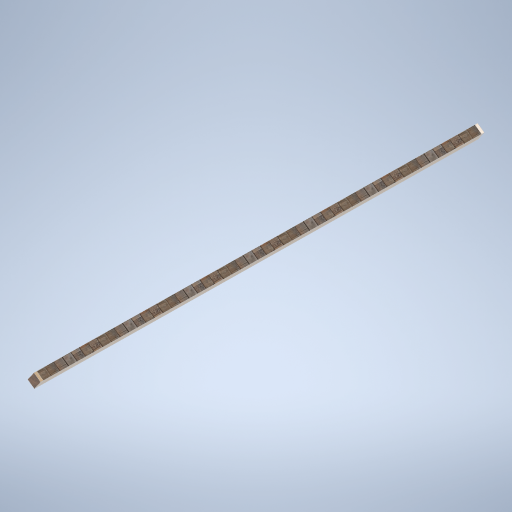
# Autodesk Inventor part: support_beam_segment_0106
Saved by Autodesk Inventor 2024.2 (Build 282272000, 272)
## iProperties
Created: 2024-05-20
Part Number: support_beam_segment_0106
Material: Wood (Maple)
Document SubType Name: Modeling
Designer: LOSTER_1
Density: 0.67 g/cm^3
Appearance: Natural Maple - Glossy Dark Tint
Author: LOSTER_1
Autodesk Inventor part; units mm, degrees
ref_plane "YZ Plane" through (0, 0, 0) normal (1, 0, 0) x (0, 1, 0)
ref_plane "XZ Plane" through (0, 0, 0) normal (0, 1, 0) x (-1, 0, 0)
sketch "Sketch1" plane through (0, 0, 0) normal (0, 0, 1) x (1, 0, 0)
  line L0 (-26.862, 36.8638) -> (-141.5773, -126.9666)
  line L1 (96.5672, -49.5284) -> (-26.3079, 36.5048)
  line L2 (-141.5773, -126.9666) -> (-18.7045, -213.0031) construction
  line L3 (-18.1437, -213.3618) -> (96.5672, -49.5284)
  line L4 (96.0404, -49.1304) -> (-18.7045, -213.0031)
  line L5 (-18.7045, -213.0031) -> (-141.5773, -126.9666)
  line L6 (-141.5773, -126.9666) -> (-26.8324, 36.9061)
  line L7 (-26.8324, 36.9061) -> (96.0404, -49.1304)
  line L8 (96.0404, -49.1304) -> (-141.5773, -126.9666) construction
  line L9 (-18.7045, -213.0031) -> (-26.8324, 36.9061) construction
  point P0 (0, 0)
  point P1 (-22.7685, -88.0485)
  constraints: 20 end point, 2 midpoint, 2 parallel, 1 perpendicular
ref_plane "Work Plane2" through (0, 0, 8101) normal (0, 0, 1) x (1, 0, 0)
ref_plane "Work Plane1" through (0, 0, 0) normal (0, 0, 1) x (1, 0, 0)
sketch "Sketch2" plane through (0, 0, 8101) normal (0, 0, 1) x (1, 0, 0)
  line L0 (190.5115, 148.9161) -> (67.641, 234.9559) construction
  line L1 (67.641, 234.9559) -> (-47.0787, 71.1285) construction
  line L2 (75.7918, -14.9112) -> (190.5115, 148.9161) construction
  line L3 (-47.0787, 71.1285) -> (75.7918, -14.9112) construction
  line L4 (190.5115, 148.9161) -> (75.7918, -14.9112)
  line L5 (75.7918, -14.9112) -> (-47.0787, 71.1285)
  line L6 (-47.0787, 71.1285) -> (67.641, 234.9559)
  line L7 (67.641, 234.9559) -> (190.5115, 148.9161)
  line L8 (190.5115, 148.9161) -> (-47.0787, 71.1285) construction
  line L9 (75.7918, -14.9112) -> (67.641, 234.9559) construction
  point P0 (0, 0)
  point P1 (71.7164, 110.0223)
  constraints: 12 end point, 2 midpoint, 2 parallel, 1 perpendicular
loft "Loft1" add profiles "Sketch1", "Sketch2"
sketch "Sketch3" plane through (-18.7045, -213.0031, 0) normal (0, 0, -1) x (-0.819152, 0.5735764, 0)
  line L0 (0, 200.0516) -> (0, 0) projected
  line L1 (0, 0) -> (150, 0) projected
  line L2 (150, 0) -> (150, 200.0516) projected
  line L3 (150, 200.0516) -> (0, 200.0516) projected
  point P0 (106.8517, 185.2104)
sketch "Sketch4" plane through (75.7918, -14.9112, 8101) normal (0, 0, 1) x (0.8191367, -0.5735984, 0)
  line L0 (0, 200) -> (0, 0) construction
  line L1 (-150, 200) -> (0, 200) construction
  line L2 (-150, 0) -> (-150, 200) construction
  line L3 (0, 0) -> (-150, 0) construction
  point P0 (-70.6369, -31.2597)
extrude "Extrusion1" add sketch "Sketch3" along normal blind 50
sketch "Sketch5" plane through (75.7918, -14.9112, 8101) normal (0, 0, 1) x (0.8191367, -0.5735984, 0)
  line L0 (-150, 0) -> (-150, 200) projected
  line L1 (0, 0) -> (-150, 0) projected
  line L2 (-150, 200) -> (0, 200)
  line L3 (0, 200) -> (0, 0)
  line L4 (0, 0) -> (-150, 0)
  line L5 (-150, 0) -> (-150, 200)
  point P0 (-70.6369, -31.2597)
  constraints: 8 end point, 2 parallel, 1 horizontal, 1 perpendicular
extrude "Extrusion2" add sketch "Sketch5" along normal blind 50
body "Solid1"
